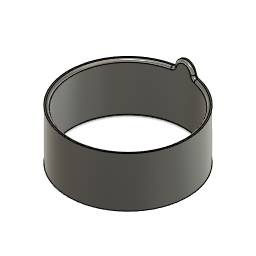
FingerGuard (Autodesk Fusion 360 design; units mm, degrees)
Autodesk Fusion 360 part; units mm, degrees
note: some values were not read from the file. Chosen so that the rebuilt part matches the saved one: which face or edge a step refers to. Set by a fixed rule: which sketch regions a step uses.
sketch "Sketch1" plane through (0, 0, 0) normal (0, 1, 0) x (1, 0, 0)
  ellipse E0 centre (0, 0) end of major axis (0, 11.17) minor radius 11.17
  line L0 (0, -11.17) -> (0, 11.17)
  line L1 (11.17, 0) -> (-11.17, 0)
  circle A0 centre (0, 0) radius 11.92
  dimension "d6" = 22.34
  dimension "d7" = 22.34
  dimension "d23" = 0.75
  constraint coincident E0.centre A0.centre
  constraint vertical L0
  constraint coincident E0 L0.start
  constraint coincident E0 L0.end
  constraint coincident E0 L1.start
  constraint coincident E0 L1.end
  measures "d6" distance of E0
  measures "d7" distance of E0
extrude "Extrude1" add sketch "Sketch1" along normal blind 12
ref_plane "WorkPlane1" through (0, 0, 11.92) normal (0, 0, 1) x (1, 0, 0)
sketch "Sketch2" plane through (0, 0, 11.92) normal (0, 0, 1) x (1, 0, 0)
  line L0 (0, 0) -> (0, 12) construction
  line L1 (0, 12) -> (-11.92, 12)
  line L2 (0, 12) -> (-11.92, 12)
  line L3 (-11.92, 12) -> (-11.92, 10)
  line L4 (-11.92, 10) -> (0, 10)
  line L5 (0, 10) -> (0, 12)
  circle A0 centre (0, 10) radius 2
  line L6 (0, 12) -> (11.92, 12)
  line L7 (11.92, 12) -> (11.92, 10)
  line L8 (11.92, 10) -> (0, 10)
  circle A1 centre (0, 10) radius 2
  dimension "d11" = 12
  dimension "d12" = 11.92
  dimension "d13" = 11.92
  dimension "d14" = 2
  constraint vertical L0
  constraint coincident L0.start origin
  constraint perpendicular L0 L1
  constraint horizontal L2
  constraint vertical L3
  constraint horizontal L4
  constraint vertical L5
  constraint coincident L4.end L5.start
  constraint coincident L0.end A0
  constraint symmetric L1.start L0 L2.start
  constraint symmetric L0 L1.end L6.end
  constraint symmetric L0 L3.end L7.end
  constraint symmetric L0 L4.end L5.start
  constraint symmetric L0 A0 A1
  measures "d11" distance of L0.start L0.end
  measures "d12" distance of L0.end L1.end
  measures "d13" distance of L0.end L1.end
  measures "d14" distance of L0.end L4.end
extrude "Extrude2" cut sketch "Sketch2" against normal blind 23.84 contours L1 L2 L3 L4 A0 A1 | A0 L6 L7 L8 A1
extrude "Extrude3" cut sketch "Sketch2" against normal blind 9 contours L5 A0 L8 A1 | L4 L5 A0 A1
fillet "Fillet1" radius 0.5 10 edges at (2, 10, -11.3703) (8.5764, 10, -7.1564) (8.5766, 10, 7.1562) (1.0041, 10, 11.1248) (-1.0041, 10, 11.1248) (-8.5764, 10, 7.1564) (-8.5764, 10, -7.1564) (-2, 10, -11.3703) (-1.5101, 11.3113, -11.0675) (1.51, 11.3114, -11.0675)
fillet "Fillet2" radius 0.5 4 edges at (-7.8984, 0, -7.8984) (-7.8984, 0, 7.8984) (7.8984, 0, 7.8984) (7.8984, 0, -7.8984)
equation "x_dim = 22.34 mm"
equation "y_dim = 10 mm"
equation "z_dim = 22.34 mm"
equation "Thickness = 0.75 mm"
equation "Swoop = 2 mm"
equation "d6 = z_dim"
equation "d7 = x_dim"
equation "d8 = y_dim + Swoop"
equation "d10 = z_dim / 2 + Thickness"
equation "d11 = y_dim + Swoop"
equation "d12 = x_dim / 2 + Thickness"
equation "d13 = x_dim / 2 + Thickness"
equation "d14 = Swoop"
equation "d15 = -( z_dim + 2 * Thickness )"
equation "d23 = Thickness"
